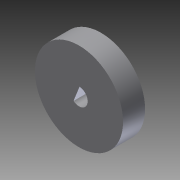
# Autodesk Inventor part: smallGearBearingBlock
Saved by Autodesk Inventor 2012 (Build 160160000, 160)
## iProperties
Created: 2014-06-12
Part Number: smallGearBearingBlock
Material: Default
Document SubType Name: Modeling
Designer: Byron
Density: 1 g/cm^3
Author: Byron
Autodesk Inventor part; units mm, degrees
ref_plane "YZ Plane" through (0, 0, 0) normal (1, 0, 0) x (0, 1, 0)
ref_plane "XZ Plane" through (0, 0, 0) normal (0, 1, 0) x (-1, 0, 0)
ref_plane "XY Plane" through (0, 0, 0) normal (0, 0, 1) x (1, 0, 0)
sketch "Sketch1" plane through (0, 0, 0) normal (0, 0, 1) x (1, 0, 0)
  line L0 (-1.579, -1.9382) -> (0.1616, 2.4948) projected
  arc A0 (-1.579, -1.9382) -> (0.1616, 2.4948) centre (0, 0) ccw projected
  arc A1 (8.0152, 21.2958) -> (7.9877, 26.3318) centre (-11.0232, 23.7099) ccw projected
  arc A2 (7.9877, 26.3318) -> (6.2484, 26.7978) centre (0, 0) ccw projected
  arc A3 (6.2484, 26.7978) -> (3.7066, 22.4502) centre (21.4014, 15.0218) ccw projected
  arc A4 (3.7066, 22.4502) -> (2.2303, 22.6446) centre (0, 0) ccw projected
  arc A5 (2.2303, 22.6446) -> (0.9003, 27.5019) centre (-16.7842, 20.049) ccw projected
  arc A6 (0.9003, 27.5019) -> (-0.9003, 27.5019) centre (0, 0) ccw projected
  arc A7 (-0.9003, 27.5019) -> (-2.2303, 22.6446) centre (16.7842, 20.049) ccw projected
  arc A8 (-2.2303, 22.6446) -> (-3.7066, 22.4502) centre (0, 0) ccw projected
  arc A9 (-3.7066, 22.4502) -> (-6.2484, 26.7978) centre (-21.4014, 15.0218) ccw projected
  arc A10 (-6.2484, 26.7978) -> (-7.9877, 26.3318) centre (0, 0) ccw projected
  arc A11 (-7.9877, 26.3318) -> (-8.0152, 21.2958) centre (11.0232, 23.7099) ccw projected
  arc A12 (-8.0152, 21.2958) -> (-9.3908, 20.7259) centre (0, 0) ccw projected
  arc A13 (-9.3908, 20.7259) -> (-12.9713, 24.2675) centre (-24.5601, 8.9709) ccw projected
  arc A14 (-12.9713, 24.2675) -> (-14.5307, 23.3672) centre (0, 0) ccw projected
  arc A15 (-14.5307, 23.3672) -> (-13.2538, 18.4956) centre (4.511, 25.7551) ccw projected
  arc A16 (-13.2538, 18.4956) -> (-14.4351, 17.5892) centre (0, 0) ccw projected
  arc A17 (-14.4351, 17.5892) -> (-18.8102, 20.0834) centre (-26.045, 2.3086) ccw projected
  arc A18 (-18.8102, 20.0834) -> (-20.0834, 18.8102) centre (0, 0) ccw projected
  arc A19 (-20.0834, 18.8102) -> (-17.5892, 14.4351) centre (-2.3086, 26.045) ccw projected
  arc A20 (-17.5892, 14.4351) -> (-18.4956, 13.2538) centre (0, 0) ccw projected
  arc A21 (-18.4956, 13.2538) -> (-23.3672, 14.5307) centre (-25.7551, -4.511) ccw projected
  arc A22 (-23.3672, 14.5307) -> (-24.2675, 12.9713) centre (0, 0) ccw projected
  arc A23 (-24.2675, 12.9713) -> (-20.7259, 9.3908) centre (-8.9709, 24.5601) ccw projected
  arc A24 (-20.7259, 9.3908) -> (-21.2958, 8.0152) centre (0, 0) ccw projected
  arc A25 (-21.2958, 8.0152) -> (-26.3318, 7.9877) centre (-23.7099, -11.0232) ccw projected
  arc A26 (-26.3318, 7.9877) -> (-26.7978, 6.2484) centre (0, 0) ccw projected
  arc A27 (-26.7978, 6.2484) -> (-22.4502, 3.7066) centre (-15.0218, 21.4014) ccw projected
  arc A28 (-22.4502, 3.7066) -> (-22.6446, 2.2303) centre (0, 0) ccw projected
  arc A29 (-22.6446, 2.2303) -> (-27.5019, 0.9003) centre (-20.049, -16.7842) ccw projected
  arc A30 (-27.5019, 0.9003) -> (-27.5019, -0.9003) centre (0, 0) ccw projected
  arc A31 (-27.5019, -0.9003) -> (-22.6446, -2.2303) centre (-20.049, 16.7842) ccw projected
  arc A32 (-22.6446, -2.2303) -> (-22.4502, -3.7066) centre (0, 0) ccw projected
  arc A33 (-22.4502, -3.7066) -> (-26.7978, -6.2484) centre (-15.0218, -21.4014) ccw projected
  arc A34 (-26.7978, -6.2484) -> (-26.3318, -7.9877) centre (0, 0) ccw projected
  arc A35 (-26.3318, -7.9877) -> (-21.2958, -8.0152) centre (-23.7099, 11.0232) ccw projected
  arc A36 (-21.2958, -8.0152) -> (-20.7259, -9.3908) centre (0, 0) ccw projected
  arc A37 (-20.7259, -9.3908) -> (-24.2675, -12.9713) centre (-8.9709, -24.5601) ccw projected
  arc A38 (-24.2675, -12.9713) -> (-23.3672, -14.5307) centre (0, 0) ccw projected
  arc A39 (-23.3672, -14.5307) -> (-18.4956, -13.2538) centre (-25.7551, 4.511) ccw projected
  arc A40 (-18.4956, -13.2538) -> (-17.5892, -14.4351) centre (0, 0) ccw projected
  arc A41 (-17.5892, -14.4351) -> (-20.0834, -18.8102) centre (-2.3086, -26.045) ccw projected
  arc A42 (-20.0834, -18.8102) -> (-18.8102, -20.0834) centre (0, 0) ccw projected
  arc A43 (-18.8102, -20.0834) -> (-14.4351, -17.5892) centre (-26.045, -2.3086) ccw projected
  arc A44 (-14.4351, -17.5892) -> (-13.2538, -18.4956) centre (0, 0) ccw projected
  arc A45 (-13.2538, -18.4956) -> (-14.5307, -23.3672) centre (4.511, -25.7551) ccw projected
  arc A46 (-14.5307, -23.3672) -> (-12.9713, -24.2675) centre (0, 0) ccw projected
  arc A47 (-12.9713, -24.2675) -> (-9.3908, -20.7259) centre (-24.5601, -8.9709) ccw projected
  arc A48 (-9.3908, -20.7259) -> (-8.0152, -21.2958) centre (0, 0) ccw projected
  arc A49 (-8.0152, -21.2958) -> (-7.9877, -26.3318) centre (11.0232, -23.7099) ccw projected
  arc A50 (-7.9877, -26.3318) -> (-6.2484, -26.7978) centre (0, 0) ccw projected
  arc A51 (-6.2484, -26.7978) -> (-3.7066, -22.4502) centre (-21.4014, -15.0218) ccw projected
  arc A52 (-3.7066, -22.4502) -> (-2.2303, -22.6446) centre (0, 0) ccw projected
  arc A53 (-2.2303, -22.6446) -> (-0.9003, -27.5019) centre (16.7842, -20.049) ccw projected
  arc A54 (-0.9003, -27.5019) -> (0.9003, -27.5019) centre (0, 0) ccw projected
  arc A55 (0.9003, -27.5019) -> (2.2303, -22.6446) centre (-16.7842, -20.049) ccw projected
  arc A56 (2.2303, -22.6446) -> (3.7066, -22.4502) centre (0, 0) ccw projected
  arc A57 (3.7066, -22.4502) -> (6.2484, -26.7978) centre (21.4014, -15.0218) ccw projected
  arc A58 (6.2484, -26.7978) -> (7.9877, -26.3318) centre (0, 0) ccw projected
  arc A59 (7.9877, -26.3318) -> (8.0152, -21.2958) centre (-11.0232, -23.7099) ccw projected
  arc A60 (8.0152, -21.2958) -> (9.3908, -20.7259) centre (0, 0) ccw projected
  arc A61 (9.3908, -20.7259) -> (12.9713, -24.2675) centre (24.5601, -8.9709) ccw projected
  arc A62 (12.9713, -24.2675) -> (14.5307, -23.3672) centre (0, 0) ccw projected
  arc A63 (14.5307, -23.3672) -> (13.2538, -18.4956) centre (-4.511, -25.7551) ccw projected
  arc A64 (13.2538, -18.4956) -> (14.4351, -17.5892) centre (0, 0) ccw projected
  arc A65 (14.4351, -17.5892) -> (18.8102, -20.0834) centre (26.045, -2.3086) ccw projected
  arc A66 (18.8102, -20.0834) -> (20.0834, -18.8102) centre (0, 0) ccw projected
  arc A67 (20.0834, -18.8102) -> (17.5892, -14.4351) centre (2.3086, -26.045) ccw projected
  arc A68 (17.5892, -14.4351) -> (18.4956, -13.2538) centre (0, 0) ccw projected
  arc A69 (18.4956, -13.2538) -> (23.3672, -14.5307) centre (25.7551, 4.511) ccw projected
  arc A70 (23.3672, -14.5307) -> (24.2675, -12.9713) centre (0, 0) ccw projected
  arc A71 (24.2675, -12.9713) -> (20.7259, -9.3908) centre (8.9709, -24.5601) ccw projected
  arc A72 (20.7259, -9.3908) -> (21.2958, -8.0152) centre (0, 0) ccw projected
  arc A73 (21.2958, -8.0152) -> (26.3318, -7.9877) centre (23.7099, 11.0232) ccw projected
  arc A74 (26.3318, -7.9877) -> (26.7978, -6.2484) centre (0, 0) ccw projected
  arc A75 (26.7978, -6.2484) -> (22.4502, -3.7066) centre (15.0218, -21.4014) ccw projected
  arc A76 (22.4502, -3.7066) -> (22.6446, -2.2303) centre (0, 0) ccw projected
  arc A77 (22.6446, -2.2303) -> (27.5019, -0.9003) centre (20.049, 16.7842) ccw projected
  arc A78 (27.5019, -0.9003) -> (27.5019, 0.9003) centre (0, 0) ccw projected
  arc A79 (27.5019, 0.9003) -> (22.6446, 2.2303) centre (20.049, -16.7842) ccw projected
  arc A80 (22.6446, 2.2303) -> (22.4502, 3.7066) centre (0, 0) ccw projected
  arc A81 (22.4502, 3.7066) -> (26.7978, 6.2484) centre (15.0218, 21.4014) ccw projected
  arc A82 (26.7978, 6.2484) -> (26.3318, 7.9877) centre (0, 0) ccw projected
  arc A83 (26.3318, 7.9877) -> (21.2958, 8.0152) centre (23.7099, -11.0232) ccw projected
  arc A84 (21.2958, 8.0152) -> (20.7259, 9.3908) centre (0, 0) ccw projected
  arc A85 (20.7259, 9.3908) -> (24.2675, 12.9713) centre (8.9709, 24.5601) ccw projected
  arc A86 (24.2675, 12.9713) -> (23.3672, 14.5307) centre (0, 0) ccw projected
  arc A87 (23.3672, 14.5307) -> (18.4956, 13.2538) centre (25.7551, -4.511) ccw projected
  arc A88 (18.4956, 13.2538) -> (17.5892, 14.4351) centre (0, 0) ccw projected
  arc A89 (17.5892, 14.4351) -> (20.0834, 18.8102) centre (2.3086, 26.045) ccw projected
  arc A90 (20.0834, 18.8102) -> (18.8102, 20.0834) centre (0, 0) ccw projected
  arc A91 (18.8102, 20.0834) -> (14.4351, 17.5892) centre (26.045, 2.3086) ccw projected
  arc A92 (14.4351, 17.5892) -> (13.2538, 18.4956) centre (0, 0) ccw projected
  arc A93 (13.2538, 18.4956) -> (14.5307, 23.3672) centre (-4.511, 25.7551) ccw projected
  arc A94 (14.5307, 23.3672) -> (12.9713, 24.2675) centre (0, 0) ccw projected
  arc A95 (12.9713, 24.2675) -> (9.3908, 20.7259) centre (24.5601, 8.9709) ccw projected
  arc A96 (9.3908, 20.7259) -> (8.0152, 21.2958) centre (0, 0) ccw projected
  circle A97 centre (0, 0) radius 12.7
  point P0 (0, 0)
  dimension "d0" = 25.4
  constraints: 1 centre point, 1 coincident
  measures "d0" diameter of A97
extrude "Extrusion1" add sketch "Sketch1" along normal blind 6.35 contours A97
body "Solid1"
